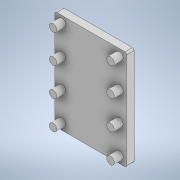
# Autodesk Inventor part: BasePlateV1
Saved by Autodesk Inventor 2022 (Build 260153000, 153)
## iProperties
Created: 2022-01-24
Part Number: BasePlateV1
Material: Generic
Document SubType Name: Modeling
Designer: money
Density: 1 g/cm^3
Appearance: Default
Author: money
Autodesk Inventor part; units mm, degrees
ref_plane "YZ Plane" through (0, 0, 0) normal (1, 0, 0) x (0, 1, 0)
ref_plane "XZ Plane" through (0, 0, 0) normal (0, 1, 0) x (-1, 0, 0)
ref_plane "XY Plane" through (0, 0, 0) normal (0, 0, 1) x (1, 0, 0)
sketch "Sketch1" plane through (0, 0, 0) normal (0, 0, 1) x (1, 0, 0)
  line L0 (3.175, 0) -> (63.5, 0)
  line L1 (25.4, 150.495) -> (0, 150.495)
  line L2 (0, 150.495) -> (0, 3.175)
  line L3 (3.175, 0) -> (25.4, 0)
  line L4 (25.4, 0) -> (25.4, 25.4)
  line L5 (25.4, 25.4) -> (0, 25.4)
  line L6 (0, 25.4) -> (0, 3.175)
  circle A0 centre (12.7, 12.7) radius 6.604
  line L7 (25.4, 25.4) -> (25.4, 50.8)
  line L8 (25.4, 50.8) -> (0, 50.8)
  line L9 (0, 50.8) -> (0, 76.835)
  line L10 (0, 76.835) -> (25.4, 76.835)
  line L11 (25.4, 76.835) -> (25.4, 50.8)
  line L12 (25.4, 76.835) -> (25.4, 102.235)
  line L13 (25.4, 102.235) -> (0, 102.235)
  line L14 (0, 102.235) -> (25.4, 102.235)
  line L15 (25.4, 102.235) -> (25.4, 127.635)
  line L16 (25.4, 127.635) -> (0, 127.635)
  line L17 (0, 127.635) -> (0, 102.235)
  line L18 (25.4, 127.635) -> (25.4, 150.495)
  circle A1 centre (12.7, 63.5) radius 6.604
  circle A2 centre (12.7, 114.3) radius 6.604
  line L19 (0, 150.495) -> (25.4, 150.495)
  line L20 (25.4, 150.495) -> (25.4, 175.895)
  line L21 (25.4, 175.895) -> (3.175, 175.895)
  line L22 (0, 172.72) -> (0, 150.495)
  circle A3 centre (12.7, 165.1) radius 6.604
  line L23 (123.825, 0) -> (63.5, 0)
  line L24 (101.6, 152.4) -> (127, 152.4)
  line L25 (127, 152.4) -> (127, 3.175)
  line L26 (123.825, 0) -> (101.6, 0)
  line L27 (101.6, 0) -> (101.6, 25.4)
  line L28 (101.6, 25.4) -> (127, 25.4)
  line L29 (127, 25.4) -> (127, 3.175)
  circle A4 centre (114.3, 12.7) radius 6.604
  line L30 (101.6, 25.4) -> (101.6, 50.8)
  line L31 (101.6, 50.8) -> (127, 50.8)
  line L32 (127, 50.8) -> (127, 76.2)
  line L33 (127, 76.2) -> (101.6, 76.2)
  line L34 (101.6, 76.2) -> (101.6, 50.8)
  line L35 (101.6, 76.2) -> (101.6, 101.6)
  line L36 (101.6, 101.6) -> (127, 101.6)
  line L37 (127, 101.6) -> (101.6, 101.6)
  line L38 (101.6, 101.6) -> (101.6, 127)
  line L39 (101.6, 127) -> (127, 127)
  line L40 (127, 127) -> (127, 101.6)
  line L41 (101.6, 127) -> (101.6, 152.4)
  circle A5 centre (114.3, 63.5) radius 6.604
  circle A6 centre (114.3, 114.3) radius 6.604
  line L42 (127, 152.4) -> (101.6, 152.4)
  line L43 (101.6, 152.4) -> (101.6, 175.895)
  line L44 (101.6, 175.895) -> (123.825, 175.895)
  line L45 (127, 172.72) -> (127, 152.4)
  circle A7 centre (114.3, 165.1) radius 6.604
  arc A8 (3.175, 175.895) -> (0, 172.72) centre (3.175, 172.72) ccw
  line L46 (25.4, 175.895) -> (101.6, 175.895)
  arc A9 (127, 172.72) -> (123.825, 175.895) centre (123.825, 172.72) ccw
  arc A10 (123.825, 0) -> (127, 3.175) centre (123.825, 3.175) ccw
  arc A11 (0, 3.175) -> (3.175, 0) centre (3.175, 3.175) ccw
  point P0 (0, 0)
  point P1 (0, 175.895)
  dimension "d3" = 25.4
  dimension "d4" = 25.4
  dimension "d5" = 13.208
  dimension "d6" = 25.4
  dimension "d7" = 25.4
  dimension "d8" = 25.4
  dimension "d9" = 25.4
  dimension "d10" = 13.208
  dimension "d11" = 13.208
  dimension "d12" = 25.4
  dimension "d13" = 25.4
  dimension "d14" = 13.208
  dimension "d15" = 3.175
  dimension "d16" = 3.175
  dimension "d17" = 3.175
  constraints: 94 end point, 12 centre point, 9 parallel, 8 point on circle, 8 tangent, 6 horizontal, 6 perpendicular, 6 point on line, 2 vertical, 1 equal radius, 1 midpoint
  measures "d3" distance of L3.end L4.end
  measures "d4" distance of L4.end L5.end
  measures "d5" diameter of A0
  measures "d6" distance of L4.end L7.end
  measures "d7" distance of L10.end L12.end
  measures "d8" distance of L15.end L16.end
  measures "d9" distance of L14.end L15.end
  measures "d10" diameter of A1
  measures "d11" diameter of A2
  measures "d12" distance of L1.start L20.end
  measures "d13" distance of L20.end point (0, 175.895)
  measures "d14" diameter of A3
  measures "d15" radius of A8
  measures "d16" radius of A9
  measures "d17" radius of A11
extrude "Extrusion1" add sketch "Sketch1" along normal blind 13.208
sketch "Sketch2" plane through (0, 0, 0) normal (0, 0, 1) x (1, 0, 0)
  circle A0 centre (12.7, 165.1) radius 6.604 projected
  circle A1 centre (12.7, 165.1) radius 6.604
  circle A2 centre (12.7, 114.3) radius 6.604 projected
  circle A3 centre (12.7, 114.3) radius 6.604
  circle A4 centre (12.7, 63.5) radius 6.604 projected
  circle A5 centre (12.7, 63.5) radius 6.604
  circle A6 centre (12.7, 12.7) radius 6.604 projected
  circle A7 centre (12.7, 12.7) radius 6.604
  circle A8 centre (114.3, 12.7) radius 6.604 projected
  circle A9 centre (114.3, 12.7) radius 6.604
  circle A10 centre (114.3, 63.5) radius 6.604 projected
  circle A11 centre (114.3, 63.5) radius 6.604
  circle A12 centre (114.3, 114.3) radius 6.604 projected
  circle A13 centre (114.3, 114.3) radius 6.604
  circle A14 centre (114.3, 165.1) radius 6.604 projected
  circle A15 centre (114.3, 165.1) radius 6.604
  point P0 (0, 0)
  constraints: 8 centre point, 8 coincident
extrude "Extrusion2" add sketch "Sketch2" along normal blind 29.083
sketch "Sketch3" plane through (0, 0, 0) normal (0, 0, 1) x (1, 0, 0)
  point P0 (0, 0)
body "Solid1"
